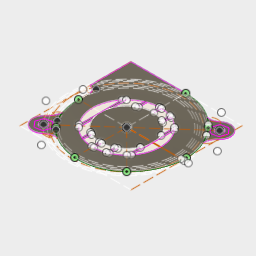
Fan Cover (Autodesk Fusion 360 design; units mm, degrees)
Autodesk Fusion 360 part; units mm, degrees
sketch "Fan Sketch" plane through (0, 0, 0) normal (0, 0, 1) x (1, 0, 0)
  circle A0 centre (60.0109, 54.7) radius 15.7
  circle A1 centre (60.0109, 54.7) radius 15.7
  line L0 (60.0109, 54.7) -> (60.0109, 70.4) construction
  line L1 (60.0109, 54.7) -> (75.7109, 54.7) construction
  line L2 (60.0109, 54.7) -> (60.0109, 39) construction
  line L3 (60.0109, 54.7) -> (44.3109, 54.7) construction
  line L4 (60.0109, 70.4) -> (60.0109, 82.1) construction
  line L5 (75.7109, 54.7) -> (86.0609, 54.7) construction
  line L6 (60.0109, 39) -> (60.0109, 30.65) construction
  line L7 (44.3109, 54.7) -> (37.6609, 54.7) construction
  line L8 (60.0109, 82.1) -> (34.6109, 82.1)
  line L9 (34.6109, 82.1) -> (34.6109, 30.65) construction
  line L10 (34.6109, 30.65) -> (86.0609, 30.65) construction
  line L11 (86.0609, 30.65) -> (86.0609, 82.1) construction
  line L12 (60.0109, 82.1) -> (86.0609, 82.1) construction
  line L13 (34.6109, 82.1) -> (34.6109, 62.9)
  line L14 (37.6609, 54.7) -> (37.6609, 62.9) construction
  line L15 (34.6109, 62.9) -> (37.6609, 62.9) construction
  arc A2 (34.6109, 62.9) -> (37.6609, 59.85) centre (37.6609, 62.9) ccw construction
  arc A3 (37.6609, 59.85) -> (34.6109, 62.9) centre (34.6109, 59.85) ccw
  line L16 (37.6609, 59.85) -> (37.6609, 54.7)
  circle A4 centre (60.0109, 54.7) radius 22.35 construction
  circle A5 centre (60.0109, 54.7) radius 24.05 construction
  circle A6 centre (60.0109, 54.7) radius 26.05 construction
  circle A7 centre (60.0109, 54.7) radius 27.4 construction
  circle A8 centre (60.0109, 54.7) radius 23.2 construction
  circle A9 centre (60.0109, 54.7) radius 25.05 construction
  circle A10 centre (60.0109, 54.7) radius 26.725 construction
  line L17 (60.0109, 54.7) -> (77.7369, 37) construction
  spline S0 degree 5 poles (37.6609, 54.7) (37.671, 53.8969) (37.7391, 52.3115) (37.9847, 49.996) (38.6041, 47.0389) (39.8862, 43.5905) (41.6938, 40.4344) (44.0279, 37.6219) (46.8577, 35.2057) (50.1114, 33.235) (53.6914, 31.7555) (57.4846, 30.8102) (61.3744, 30.4377) (65.2537, 30.6735) (69.0307, 31.5464) (72.6235, 33.0703) (75.9554, 35.2357) (78.9512, 38.0025) (81.5318, 41.2888) (83.6149, 44.9716) (85.1252, 48.9079) (86.0038, 52.9506) (86.2166, 56.9661) (85.7654, 60.8523) (84.6945, 64.5526) (83.0718, 68.0356) (80.9726, 71.2792) (78.4636, 74.2538) (75.5845, 76.9031) (72.3367, 79.1338) (68.6989, 80.8386) (65.4509, 81.6994) (62.8116, 82.0272) (60.9599, 82.1) (60.0109, 82.1) knots 0 0 0 0 0 0 0.033333 0.066667 0.1 0.133333 0.166667 0.2 0.233333 0.266667 0.3 0.333333 0.366667 0.4 0.433333 0.466667 0.5 0.533333 0.566667 0.6 0.633333 0.666667 0.7 0.733333 0.766667 0.8 0.833333 0.866667 0.9 0.933333 0.966667 1 1 1 1 1 1
  line L18 (71.0219, 82.1) -> (49, 82.1)
  line L19 (37.5312, 65.0367) -> (37.7907, 44.3632)
  line L20 (60.0109, 54.7) -> (75.7109, 54.7) construction
  circle A11 centre (60.0109, 54.7) radius 12.15
  line L21 (47.8609, 54.7) -> (47.8609, 64.6432)
  line L22 (47.8609, 54.7) -> (47.8609, 44.7568)
  line L23 (48.8609, 65.7529) -> (48.8609, 59.527)
  line L24 (48.8609, 43.6471) -> (48.8609, 49.873)
  line L25 (59.5109, 42.5608) -> (59.5109, 39.008)
  line L26 (59.5109, 70.392) -> (59.5109, 66.8397)
  line L27 (54.6859, 43.7791) -> (54.6859, 39.9306)
  line L28 (53.6859, 44.3261) -> (53.6859, 40.3304)
  line L29 (54.6859, 65.6209) -> (54.6859, 69.4694)
  line L30 (53.6859, 65.0739) -> (53.6859, 69.0696)
  line L31 (72.1609, 54.7) -> (72.1609, 64.6432)
  line L32 (71.1609, 65.7529) -> (71.1609, 59.527)
  line L33 (66.3359, 65.0739) -> (66.3359, 69.0696)
  line L34 (65.3359, 65.6209) -> (65.3359, 69.4694)
  line L35 (60.5109, 70.392) -> (60.5109, 66.8397)
  line L36 (72.1609, 54.7) -> (72.1609, 44.7568)
  line L37 (71.1609, 43.6471) -> (71.1609, 49.873)
  line L38 (66.3359, 44.3261) -> (66.3359, 40.3304)
  line L39 (65.3359, 43.7791) -> (65.3359, 39.9306)
  line L40 (60.5109, 42.5608) -> (60.5109, 39.008)
  line L41 (60.0109, 54.7) -> (86.6909, 54.7) construction
  line L42 (60.0109, 54.7) -> (88.6109, 54.7) construction
  circle A12 centre (60.0109, 54.7) radius 25.2 construction
  line L43 (60.0109, 54.7) -> (85.2109, 54.7) construction
  line L44 (82.8188, 74.9497) -> (39.5961, 36.5748) construction
  circle A13 centre (82.8188, 74.9497) radius 1.75
  circle A14 centre (39.5961, 36.5748) radius 1.75
  line L45 (40.6895, 39.8618) -> (37.2961, 39.1653)
  line L46 (37.2961, 39.1653) -> (36.2027, 35.8783)
  line L47 (36.2027, 35.8783) -> (38.5026, 33.2878)
  line L48 (38.5026, 33.2878) -> (41.896, 33.9844)
  line L49 (41.896, 33.9844) -> (42.9894, 37.2714)
  line L50 (42.9894, 37.2714) -> (40.6895, 39.8618)
  line L51 (81.7253, 71.6627) -> (85.1187, 72.3593)
  line L52 (85.1187, 72.3593) -> (86.2121, 75.6463)
  line L53 (86.2121, 75.6463) -> (83.9122, 78.2367)
  line L54 (83.9122, 78.2367) -> (80.5189, 77.5402)
  line L55 (80.5189, 77.5402) -> (79.4254, 74.2532)
  line L56 (79.4254, 74.2532) -> (81.7253, 71.6627)
  line L57 (39.5961, 36.5748) -> (36.2764, 40.3138) construction
  line L58 (39.5961, 36.5748) -> (42.9157, 32.8358) construction
  line L59 (82.8188, 74.9497) -> (86.1384, 71.2108) construction
  line L60 (82.8188, 74.9497) -> (79.4992, 78.6887) construction
  arc A15 (39.1103, 45.9033) -> (36.2764, 40.3138) centre (41.3317, 41.2639) ccw construction
  arc A16 (42.9157, 32.8358) -> (48.3213, 34.4078) centre (44.5371, 37.3402) ccw construction
  arc A17 (79.4992, 78.6887) -> (74.5478, 77.5144) centre (77.8237, 74.7276) ccw construction
  arc A18 (83.914, 66.0571) -> (86.1384, 71.2108) centre (81.6649, 70.0847) ccw construction
  line L61 (79.4992, 78.6887) -> (76.4619, 75.9921) construction
  line L62 (86.1384, 71.2108) -> (82.8006, 68.2473) construction
  arc A19 (74.5478, 77.5144) -> (79.4992, 78.6887) centre (75.931, 82.7076) ccw
  arc A20 (86.1384, 71.2108) -> (83.914, 66.0571) centre (90.5386, 66.2547) ccw
  line L63 (36.2764, 40.3138) -> (39.1103, 45.9033) construction
  line L64 (42.9157, 32.8358) -> (48.3213, 34.4078) construction
  line L65 (41.3317, 41.2639) -> (36.7439, 43.5899) construction
  line L66 (44.5371, 37.3402) -> (45.874, 32.7433) construction
  line L67 (42.9157, 32.8358) -> (46.2842, 35.8265) construction
  line L68 (36.2764, 40.3138) -> (40.0269, 43.6436) construction
  arc A21 (36.2764, 40.3138) -> (39.1103, 45.9033) centre (30.604, 46.7028) ccw
  arc A22 (48.3213, 34.4078) -> (42.9157, 32.8358) centre (47.2749, 27.9259) ccw
  arc A23 (36.2764, 40.3138) -> (42.9157, 32.8358) centre (39.5961, 36.5748) ccw
  arc A24 (86.1384, 71.2108) -> (79.4992, 78.6887) centre (82.8188, 74.9497) ccw
  point P0 (43.5943, 38.3069)
  point P1 (78.9054, 73.6004)
  point P2 (86.0609, 56.375)
  point P3 (60.0109, 54.7)
  point P4 (60.0109, 54.7)
  point P5 (60.0109, 54.7)
  point P6 (39.5961, 36.5748)
  point P7 (82.8188, 74.9497)
  dimension "d2" = 31.4
  dimension "d4" = 11.7
  dimension "d5" = 10.35
  dimension "d6" = 8.35
  dimension "d7" = 6.65
  dimension "d8" = 25.4
  dimension "d9" = 19.2
  dimension "d13" = 53.45
  dimension "d27" = 24.3
  dimension "d55" = 57.8
  dimension "d56" = 3.5
  dimension "d57" = 3.5
  dimension "d58" = 3
  dimension "d59" = 3
  measures "d2" diameter of A0
  measures "d4" distance of L0.end L4.end
  measures "d5" distance of L1.end L5.end
  measures "d6" distance of L2.end L6.end
  measures "d7" distance of L3.end L7.end
  measures "d8" distance of L4.end L8.end
  measures "d9" distance of L8.end L13.end
  measures "d13" diameter of A10
  measures "d27" diameter of A11
  measures "d55" distance of P7 P6
  measures "d56" diameter of A13
  measures "d57" diameter of A14
  measures "d58" distance of P6 L50
  measures "d59" distance of P7 L56
combine "Combine1" [no effect]
extrude "Extrude3" add sketch "Fan Sketch" along normal blind 0.2 contours A0 A1 A11 L31 L32 | A0 A1 A11 L36 L37 | A11 | A0 A1 A11 L33 L34 | A0 A1 A11 L38 L39 | A0 A1 A11 L26 L35 | A0 A1 A11 L25 L40 | A0 A1 A11 L29 L30 | A0 A1 A11 L27 L28 | A0 A1 A11 L21 L23 | A0 A1 A11 L22 L24 | L8 L13 A3 L16 S0 L18 | S0 A19 A20 A24 | S0 A21 A22 A23 | L45 L46 L47 L48 L49 L50 | L51 L52 L53 L54 L55 L56
equation "d13 = 52.100 mm + ( 11.7 mm - 10.35 mm )"
equation "d55 = 53.3 mm + 4.5 mm"
named bodies: "Fan Base"
